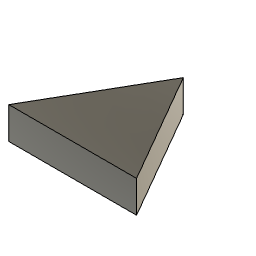
Triangle (Autodesk Fusion 360 design; units mm, degrees)
Autodesk Fusion 360 part; units mm, degrees
sketch "Triangle" plane through (0, 0, 0) normal (0, 0, 1) x (1, 0, 0)
  line L0 (0, -10.9985) -> (6.35, 0)
  line L1 (12.7, -10.9985) -> (0, -10.9985)
  line L2 (6.35, 0) -> (12.7, -10.9985)
extrude "Extrude1" add sketch "Triangle" along normal blind 3.175
